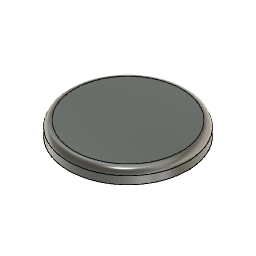
CR2025_3v_battery v1 (Autodesk Fusion 360 design; units mm, degrees)
Autodesk Fusion 360 part; units mm, degrees
sketch "Sketch1" plane through (0, 0, 0) normal (0, 0, 1) x (1, 0, 0)
  circle A0 centre (0, 0) radius 9.95
  dimension "d1" = 19.9
  constraint coincident A0.centre origin
  measures "d1" diameter of A0
extrude "Extrude1" add sketch "Sketch1" along normal blind 2.3
fillet "Fillet1" radius 1 1 faces at (-3.1693, 3.5342, 2.3)
sketch "Sketch2" plane through (0, 0, 2.3) normal (0, 0, 1) x (-1, 0, 0)
  circle A0 centre (0, 0) radius 8.95
